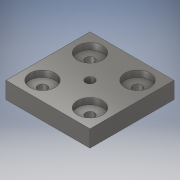
# Autodesk Inventor part: feet type 1 part 1
Saved by Autodesk Inventor 2018 (Build 220112000, 112)
## iProperties
Created: 2018-10-16
Part Number: feet type 1 part 1
Material: Stainless Steel
Document SubType Name: Modeling
Designer: freyja
Mass: 343.87 g
Surface Area: 132.017 cm^2
Volume: 42.9837 cm^3
Density: 8 g/cm^3
Appearance: Semi-Polished
Author: freyja
Autodesk Inventor part; units mm, degrees
note: some values were not read from the file. Chosen so that the rebuilt part matches the saved one: direction of "Hole1"; direction of "Hole2".
ref_plane "YZ Plane" through (0, 0, 0) normal (1, 0, 0) x (0, 1, 0)
ref_plane "XZ Plane" through (0, 0, 0) normal (0, 1, 0) x (-1, 0, 0)
ref_plane "XY Plane" through (0, 0, 0) normal (0, 0, 1) x (1, 0, 0)
sketch "Sketch1" plane through (0, 0, 0) normal (0, 1, 0) x (-1, 0, 0)
  line L0 (-31.75, 31.75) -> (31.75, 31.75)
  line L1 (31.75, 31.75) -> (31.75, -31.75)
  line L2 (31.75, -31.75) -> (-31.75, -31.75)
  line L3 (-31.75, -31.75) -> (-31.75, 31.75)
  line L4 (-31.75, 31.75) -> (31.75, -31.75) construction
  line L5 (31.75, 31.75) -> (-31.75, -31.75) construction
  point P0 (0, 0)
  dimension "d0" = 63.5
  dimension "d1" = 63.5
  constraints: 12 end point, 2 midpoint, 2 parallel, 1 horizontal, 1 perpendicular
  measures "d0" distance of L1.end L2.end
  measures "d1" distance of L0.end L1.end
extrude "Extrusion1" add sketch "Sketch1" along normal blind 12.7
sketch "Sketch2" plane through (0, 12.7, 0) normal (0, 1, 0) x (1, 0, 0)
  line L0 (0, 0) -> (17.9605, 17.9605)
  line L1 (0, 0) -> (25.4, 0) construction
  line L2 (0, 0) -> (-17.9605, 17.9605)
  line L3 (0, 0) -> (-17.9605, -17.9605)
  line L4 (0, 0) -> (17.9605, -17.9605)
  dimension "d4" = 25.4
  dimension "d5" = 45
  dimension "d8" = 360
  constraints: 10 end point, 2 coincident, 1 equal length, 1 horizontal, 11 other
  measures "d4" distance of L0.start L0.end
  measures "d5" angle of L1 L0
hole "Hole1" at (17.9605, 12.7, 17.9605) at (-17.9605, 12.7, -17.9605) at (-17.9605, 12.7, 17.9605) at (17.9605, 12.7, -17.9605) direction (0, -1, 0) diameter 6.7564 end up to surface counterbore diameter 19.05 counterbore depth 4.7752 clearance for "Hex Head Bolt" size "1/4" standard "Ansi Unified Screw Threads"
sketch "Sketch3" plane through (0, 0, 0) normal (0, -1, 0) x (1, 0, 0)
  circle A0 centre (0, 0) radius 12.7
  dimension "d17" = 25.4
  constraints: 1 centre point, 1 coincident
  measures "d17" diameter of A0
hole "Hole2" at (0, 0, 0) direction (0, 1, 0) diameter 6.7564 end up to surface counterbore diameter 19.05 counterbore depth 4.7752 clearance for "Hex Head Bolt" size "1/4" standard "Ansi Unified Screw Threads"
body "Solid1"
